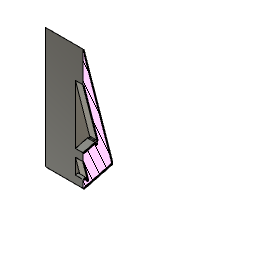
COVID-19 Vaccination Record Card Frame v3 (Autodesk Fusion 360 design; units mm, degrees)
Autodesk Fusion 360 part; units mm, degrees
sketch "Sketch1" plane through (0, 0, 0) normal (0, 0, 1) x (1, 0, 0)
  line L0 (0, 0) -> (101.6, 0)
  line L1 (101.6, 0) -> (101.6, 76.2)
  line L2 (101.6, 76.2) -> (0, 76.2)
  line L3 (0, 76.2) -> (0, 0)
  line L4 (-40, -40) -> (141.6, -40)
  line L5 (141.6, -40) -> (141.6, 116.2)
  line L6 (141.6, 116.2) -> (-40, 116.2)
  line L7 (-40, 116.2) -> (-40, -40)
  line L8 (0, -30) -> (101.6, -30)
  line L9 (101.6, -30) -> (101.6, -10)
  line L10 (101.6, -10) -> (0, -10)
  line L11 (0, -10) -> (0, -30)
  dimension "d1" = 101.6
  dimension "d2" = 76.2
  dimension "frame_margin_height" = 40
  dimension "d7" = 40
  dimension "frame_margin_width" = 40
  dimension "d9" = 40
  dimension "d10" = 20
  dimension "d11" = 10
  constraint horizontal L0
  constraint vertical L1
  constraint horizontal L2
  constraint vertical L3
  constraint coincident L0.start L3.end
  constraint horizontal L4
  constraint vertical L5
  constraint horizontal L6
  constraint vertical L7
  constraint horizontal L8
  constraint vertical L9
  constraint horizontal L10
  constraint vertical L11
  constraint vertical L0.end L9.end
  constraint vertical L0.start L10.end
  measures "d1" distance of L0.start L0.end
  measures "d2" distance of L0.start L2.end
  measures "frame_margin_height" distance of L2 L6
  measures "d7" distance of L0 L4
  measures "frame_margin_width" distance of L3 L7
  measures "d9" distance of L1 L5
  measures "d10" distance of L8 L10
  measures "d11" distance of L0 L10
ref_plane "WorkPlane1" through (-40, 0, 0) normal (1, 0, 0) x (0, 1, 0)
sketch "Sketch8" plane through (-40, 0, 0) normal (1, 0, 0) x (0, 1, 0)
  line L0 (-40, 0) -> (-40, 40)
  line L1 (-40, 0) -> (116.2, 0)
  line L2 (-40, 40) -> (116.2, 0)
  point P0 (116.2, 0)
  point P1 (-40, 0)
  dimension "d18" = 40
  constraint vertical L0
  constraint perpendicular L0 L1
  constraint coincident P0 L1.end
  constraint coincident L0.start L1.start
  measures "d18" distance of L0.start L0.end
extrude "Extrude2" add sketch "Sketch8" along normal up to surface (181.6 mm away)
extrude "Extrude3" cut sketch "Sketch1" along normal up to surface contours L0 L1 L2 L3 | L8 L9 L10 L11 end surface through (-40, -40, 40) normal (0, 0.248077, 0.96874) offset 0
extrude "Extrude4" add 1 faces at (67.7333, 76.2, 3.4144) along direction (0, -1, 0) up to surface (76.2 mm away)
sketch "Sketch10" plane through (0, 0, 0) normal (1, 0, 0) x (0, 1, 0)
  line L0 (0, 10.2433) -> (76.2, 10.2433)
  line L1 (76.2, 10.2433) -> (0, 29.7567)
  line L2 (0, 29.7567) -> (0, 10.2433)
  line L3 (76.2, 10.2433) -> (0, 11.7433)
  line L4 (0, 11.7433) -> (-2.9994, 11.8023)
  line L5 (-2.9994, 11.8023) -> (-2.9699, 13.302)
  line L6 (-2.9699, 13.302) -> (0, 13.2436)
  line L7 (0, 13.2436) -> (0, 11.7433)
  dimension "d25" = 1.5
  dimension "d27" = 3
  dimension "d28" = 1.5
  constraint coincident L0.end L1.start
  constraint coincident L2 L3.end
  constraint parallel L3 L4
  constraint perpendicular L4 L5
  constraint coincident L2 L6.end
  constraint perpendicular L5 L6
  measures "d25" distance of L0.start L3.end
  measures "d27" distance of L3.end L4.end
  measures "d28" distance of L4.end L5.end
extrude "Extrude5" cut sketch "Sketch10" along normal up to surface (101.6 mm away) contours L2 L4 L5 L6 L7
extrude "Extrude6" add 1 faces at (67.7333, -10, 10.7725) along direction (0, -1, 0) up to surface (20 mm away)
sketch "Sketch11" plane through (0, 0, 0) normal (1, 0, 0) x (0, 1, 0)
  line L0 (-30, 32.3175) -> (-10, 32.3175)
  line L1 (-10, 32.3175) -> (-30, 37.4392)
  line L2 (-30, 37.4392) -> (-30, 32.3175)
  line L3 (-30, 32.3175) -> (-35, 32.3175)
  line L4 (-35, 32.3175) -> (-35, 33.8175)
  line L5 (-35, 33.8175) -> (-30, 33.8175)
  line L6 (-30, 32.3175) -> (-30, 33.8175)
  dimension "d33" = 5
  dimension "d34" = 1.5
  constraint horizontal L3
  constraint coincident L0.start L2.end
  constraint perpendicular L3 L4
  constraint coincident L2 L5.end
  constraint perpendicular L2 L5
  measures "d33" distance of L0.start L3.end
  measures "d34" distance of L3.end L4.end
extrude "Extrude7" cut sketch "Sketch11" along normal up to surface (101.6 mm away) contours L2 L3 L4 L5 L6
move_body "Move1" bodies 1 to x (1, 0, 0) y (0, 0, 1) z (0, -1, 0) at (0, 0, 80)
move_body "Move2" bodies 1 to x (1, 0, 0) y (0, 0.968583, 0.24869) z (0, -0.24869, 0.968583) at (0, 8.6909, 11.2043)
equation "d1 = cdc_card_width"
equation "d2 = cdc_card_height"
equation "cdc_card_height = 3 in"
equation "cdc_card_width = 4 in"
equation "cdc_card_thickness = 0.45 mm" comment "Includes allowable tolerance; measurements were between 0.3 and 0.45, depending on stickers"
equation "d7 = frame_margin_height"
equation "d9 = frame_margin_width"
equation "d10 = frame_margin_height / 2"
equation "d11 = frame_margin_height / 4"
named bodies: "Frame"
